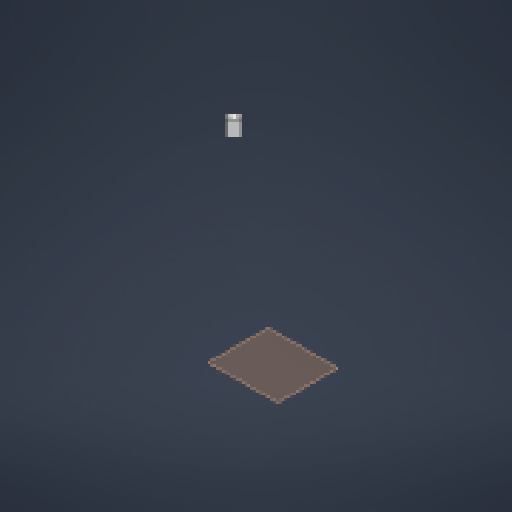
# Autodesk Inventor part: Standoff
Saved by Autodesk Inventor 2023 (Build 270158000, 158)
## iProperties
Created: 2023-02-16
Part Number: Standoff
Material: Generic
Document SubType Name: Modeling
Designer: Michael
Density: 1 g/cm^3
Appearance: Default
Author: Michael
Autodesk Inventor part; units mm, degrees
ref_plane "YZ Plane" through (0, 0, 0) normal (1, 0, 0) x (0, 1, 0)
ref_plane "XZ Plane" through (0, 0, 0) normal (0, 1, 0) x (-1, 0, 0)
ref_plane "XY Plane" through (0, 0, 0) normal (0, 0, 1) x (1, 0, 0)
ref_plane "Work Plane1" through (49.1494, -37.6525, 49.2967) normal (0, 1, 0) x (-1, 0, 0)
sketch "Sketch2" plane through (49.1494, -37.6525, 49.2967) normal (0, 1, 0) x (-1, 0, 0)
  line L0 (662.4608, -525.6919) -> (646.2945, -509.5274) projected
  line L1 (143.1429, -6.4305) -> (69.9168, -79.6645) projected
  line L2 (623.8451, -531.9793) -> (639.991, -548.1234) projected
  line L3 (104.5272, -12.7179) -> (126.9766, 9.734) projected
  line L4 (646.2945, -509.5274) -> (662.4608, -525.6919)
  line L5 (662.4608, -525.6919) -> (639.991, -548.1234)
  line L6 (639.991, -548.1234) -> (623.8451, -531.9793)
  line L7 (623.8451, -531.9793) -> (646.2945, -509.5274)
  point P0 (49.1494, -49.2967)
  point P1 (69.9168, -79.6645)
  constraints: 8 end point, 3 equal length
extrude "Extrusion2" add sketch "Sketch2" along normal blind 44.45
sketch "Sketch3" plane through (49.1494, 6.7975, 49.2967) normal (0, 1, 0) x (1, 0, 0)
  circle A0 centre (-647.1931, 521.2017) radius 2.4765 projected
  circle A1 centre (-635.5195, 532.8766) radius 2.4765 projected
  point P0 (-49.1494, 49.2967)
  constraints: 2 coincident
hole "Hole1" at (-586.3701, 6.7975, -483.58) at (-598.0438, 6.7975, -471.905) direction (0, -1, 0) diameter 7.112 depth 10.414
sketch "Sketch4" plane through (49.1494, -37.6525, 49.2967) normal (0, -1, 0) x (1, 0, 0)
  circle A0 centre (-647.1931, -521.2017) radius 3.556 projected
  circle A1 centre (-635.5195, -532.8766) radius 3.556 projected
  point P0 (-49.1494, -49.2967)
extrude "Extrusion3" cut sketch "Sketch4" against normal blind 10.414
fillet "Fillet1" radius 3.175 2 edges at (-590.8417, -15.4275, -498.8268) (-613.3114, -15.4275, -476.3953)
body "Solid2"
